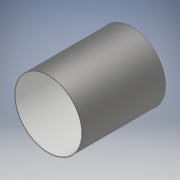
# Autodesk Inventor part: Part 2 of Focusrite Microphone
Saved by Autodesk Inventor 2018 (Build 220112000, 112)
## iProperties
Created: 2017-11-13
Part Number: Part 2 of Focusrite Microphone
Material: Generic
Document SubType Name: Modeling
Designer: Justin
Density: 1 g/cm^3
Appearance: Default
Author: Justin
Autodesk Inventor part; units mm, degrees
ref_plane "YZ Plane" through (0, 0, 0) normal (1, 0, 0) x (0, 1, 0)
ref_plane "XZ Plane" through (0, 0, 0) normal (0, 1, 0) x (-1, 0, 0)
ref_plane "XY Plane" through (0, 0, 0) normal (0, 0, 1) x (1, 0, 0)
sketch "Sketch1" plane through (0, 0, 0) normal (0, 0, 1) x (1, 0, 0)
  line L0 (0, 0) -> (28.485, 0)
  line L1 (0, 0) -> (28.485, 0) construction
  line L2 (28.485, 0) -> (28.485, 70)
  line L3 (28.485, 70) -> (27.485, 70)
  line L4 (27.485, 70) -> (27.985, 0)
  line L5 (0, 0) -> (0, 1)
  dimension "d0" = 28.485
  dimension "d1" = 0
  dimension "d2" = 70
  dimension "d3" = 1
  dimension "d4" = 1
  constraints: 12 end point, 3 perpendicular, 2 horizontal, 1 collinear, 1 point on line
  measures "d0" distance of L0.start L0.end
  measures "d1" distance between parallel lines of L0 L1
  measures "d2" distance of L0.end L2.end
  measures "d3" distance of L2.end L3.end
  measures "d4" distance of L0.start L5.end
revolve "Revolution1" add sketch "Sketch1" angle 360 about axis through (0, 0, 0) along (0, 1, 0)
body "Solid1"
